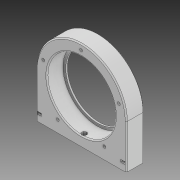
# Autodesk Inventor part: J0_drivebracket
Saved by Autodesk Inventor 2020 (Build 240168000, 168)
## iProperties
Created: 2021-03-20
Part Number: J0_drivebracket
Material: Generic
Document SubType Name: Modeling
Designer: DDeGo
Density: 1 g/cm^3
Appearance: Default
Author: DDeGo
Autodesk Inventor part; units mm, degrees
ref_plane "YZ Plane" through (0, 0, 0) normal (1, 0, 0) x (0, 1, 0)
ref_plane "XZ Plane" through (0, 0, 0) normal (0, 1, 0) x (-1, 0, 0)
ref_plane "XY Plane" through (0, 0, 0) normal (0, 0, 1) x (1, 0, 0)
sketch "Sketch1" plane through (0, 0, 0) normal (0, 0, 1) x (1, 0, 0)
  circle A0 centre (0, 0) radius 62.55
  arc A1 (82.55, 0) -> (-82.55, 0) centre (0, 0) ccw
  line L0 (-82.55, 0) -> (-82.55, -80)
  line L1 (-82.55, -80) -> (82.55, -80)
  line L2 (82.55, -80) -> (82.55, 0)
  dimension "d0" = 125.1
  dimension "d1" = 20
  dimension "d2" = 80
  constraints: 6 end point, 2 centre point, 2 coincident, 2 point on circle, 2 tangent, 2 vertical, 1 perpendicular
  measures "d0" diameter of A0
  measures "d1" radial gap between concentric circles of A1 A0
  measures "d2" distance from line of L1 point (0, 0)
extrude "Extrusion1" add sketch "Sketch1" along normal blind 32.5
sketch "Sketch2" plane through (0, 0, 0) normal (0, 0, -1) x (-1, 0, 0)
  circle A0 centre (0, 0) radius 62.55 projected
  circle A1 centre (0, 0) radius 57.55
  dimension "d5" = 5
  constraints: 1 centre point, 1 coincident
  measures "d5" radial gap between concentric circles of A0 A1
extrude "Extrusion2" add sketch "Sketch2" against normal blind 3
sketch "Sketch3" plane through (0, 0, 32.5) normal (0, 0, 1) x (1, 0, 0)
  arc A0 (82.55, 0) -> (-82.55, 0) centre (0, 0) ccw construction
  line L0 (0, 0) -> (0, 72.5) construction
  circle A1 centre (0, 72.5) radius 2.6
  circle A2 centre (-68.9516, 22.4037) radius 2.6
  circle A3 centre (-42.6144, -58.6537) radius 2.6
  circle A4 centre (42.6144, -58.6537) radius 2.6
  circle A5 centre (68.9516, 22.4037) radius 2.6
  dimension "d8" = 5.2
  dimension "d9" = 72.5
  dimension "d12" = 360
  constraints: 5 centre point, 5 coincident, 2 end point, 1 vertical, 16 other
  measures "d8" diameter of A1
  measures "d9" distance of L0.start L0.end
extrude "Extrusion3" cut sketch "Sketch3" against normal through all
sketch "Sketch5" plane through (-82.55, -80, 0) normal (0, -1, 0) x (1, 0, 0)
  circle A0 centre (6, 26.5) radius 2.75
  circle A1 centre (159.1, 26.5) radius 2.75
  circle A2 centre (120.825, 6) radius 2.75
  circle A3 centre (44.275, 6) radius 2.75
  circle A4 centre (82.55, 26.5) radius 2.75
  line L0 (6, 26.5) -> (82.55, 26.5) construction
  line L1 (82.55, 26.5) -> (159.1, 26.5) construction
  line L2 (120.825, 6) -> (44.275, 6) construction
  line L3 (82.55, 26.5) -> (82.55, 6) construction
  line L4 (82.55, 6) -> (82.55, 0) construction
  line L5 (0, 0) -> (165.1, 0) construction
  line L6 (0, 32.5) -> (165.1, 32.5) construction
  line L7 (0, 0) -> (0, 32.5) construction
  line L8 (44.275, 26.5) -> (44.275, 6) construction
  dimension "d16" = 5.5
  dimension "d17" = 6
  dimension "d18" = 6
  dimension "d19" = 6
  constraints: 12 end point, 5 centre point, 4 equal radius, 3 horizontal, 3 vertical, 2 midpoint, 1 collinear
  measures "d16" diameter of A0
  measures "d17" distance between parallel lines of L5 L2
  measures "d18" distance between parallel lines of L6 L0
  measures "d19" distance from line of L7 L0.start
extrude "Extrusion4" cut sketch "Sketch5" against normal blind 18
ref_plane "Work Plane1" through (-82.55, -64, 0) normal (0, -1, 0) x (1, 0, 0)
sketch "Sketch6" plane through (-82.55, -64, 0) normal (0, -1, 0) x (1, 0, 0)
  circle A0 centre (159.1, 26.5) radius 2.75 projected
  circle A1 centre (82.55, 26.5) radius 2.75 projected
  circle A2 centre (44.275, 6) radius 2.75 projected
  line L0 (159.1, 31.2343) -> (163.2, 28.8671) construction
  line L1 (163.2, 28.8671) -> (163.2, 24.1329)
  line L2 (163.2, 24.1329) -> (159.1, 21.7657)
  line L3 (159.1, 21.7657) -> (155, 24.1329)
  line L4 (155, 24.1329) -> (155, 28.8671)
  line L5 (155, 28.8671) -> (159.1, 31.2343) construction
  line L6 (82.55, 31.2343) -> (86.65, 28.8671)
  line L7 (86.65, 28.8671) -> (86.65, 24.1329)
  line L8 (86.65, 24.1329) -> (82.55, 21.7657)
  line L9 (82.55, 21.7657) -> (78.45, 24.1329)
  line L10 (78.45, 24.1329) -> (78.45, 28.8671)
  line L11 (78.45, 28.8671) -> (82.55, 31.2343)
  circle A3 centre (44.275, 6) radius 2.75 projected
  line L12 (44.275, 1.2657) -> (40.175, 3.6329) construction
  line L13 (40.175, 3.6329) -> (40.175, 8.3671)
  line L14 (40.175, 8.3671) -> (44.275, 10.7343)
  line L15 (44.275, 10.7343) -> (48.375, 8.3671)
  line L16 (48.375, 8.3671) -> (48.375, 3.6329)
  line L17 (48.375, 3.6329) -> (44.275, 1.2657) construction
  circle A4 centre (120.825, 6) radius 2.75 projected
  line L18 (120.825, 1.2657) -> (116.725, 3.6329) construction
  line L19 (116.725, 3.6329) -> (116.725, 8.3671)
  line L20 (116.725, 8.3671) -> (120.825, 10.7343)
  line L21 (120.825, 10.7343) -> (124.925, 8.3671)
  line L22 (124.925, 8.3671) -> (124.925, 3.6329)
  line L23 (124.925, 3.6329) -> (120.825, 1.2657) construction
  circle A5 centre (6, 26.5) radius 2.75 projected
  line L24 (6, 21.7657) -> (1.9, 24.1329)
  line L25 (1.9, 24.1329) -> (1.9, 28.8671)
  line L26 (1.9, 28.8671) -> (6, 31.2343) construction
  line L27 (6, 31.2343) -> (10.1, 28.8671) construction
  line L28 (10.1, 28.8671) -> (10.1, 24.1329)
  line L29 (10.1, 24.1329) -> (6, 21.7657)
  line L30 (163.2, 28.8671) -> (163.2, 37.0137)
  line L31 (163.2, 37.0137) -> (155, 37.0137)
  line L32 (155, 37.0137) -> (155, 28.8671)
  line L33 (124.925, 3.6329) -> (124.925, -4.8085)
  line L34 (124.925, -4.8085) -> (116.725, -4.8085)
  line L35 (116.725, -4.8085) -> (116.725, 3.6329)
  line L36 (48.375, 3.6329) -> (48.375, -5.465)
  line L37 (48.375, -5.465) -> (40.175, -5.465)
  line L38 (40.175, -5.465) -> (40.175, 3.6329)
  line L39 (20, 3) -> (145.1, 3) projected
  line L40 (10.1, 28.8671) -> (10.1, 35.0607)
  line L41 (10.1, 35.0607) -> (1.9, 35.0607)
  line L42 (1.9, 35.0607) -> (1.9, 28.8671)
  point P0 (82.55, 0)
  point P1 (6, 26.5)
  point P2 (48.375, 3)
  point P3 (40.175, 3)
  point P4 (124.925, 3)
  point P5 (116.725, 3)
  dimension "d23" = 8.2
  constraints: 84 end point, 9 vertical, 5 coincident, 5 perpendicular, 4 parallel, 3 collinear, 65 other
  measures "d23" distance between parallel lines of L4 L1
extrude "Extrusion5" cut sketch "Sketch6" along normal blind 4.5 contours A1 | L1 L2 L3 L4 L32 L31 L30 | L6 L7 L8 L9 L10 L11 | L13 L14 L15 L16 L36 L39 L38 | L39 L36 L37 L38 | L19 L20 L21 L22 L33 L39 L35 | L39 L33 L34 L35 | L24 L25 L42 L41 L40 L28 L29
extrude "Extrusion6" cut sketch "Sketch6" against normal blind 20.75 contours L6 L7 L8 L9 L10 L11
fillet "Fillet1" radius 2 1 edges at (-62.55, 0, 32.5)
chamfer "Chamfer1" distance 2 angle 45 6 edges at (0, 82.55, 32.5) (-82.55, -40, 32.5) (82.55, -40, 32.5) (0, 82.55, 0) (-82.55, -40, 0) (82.55, -40, 0)
equation "\"d18\" = d17"
equation "\"d19\" = d17"
body "Solid1"
